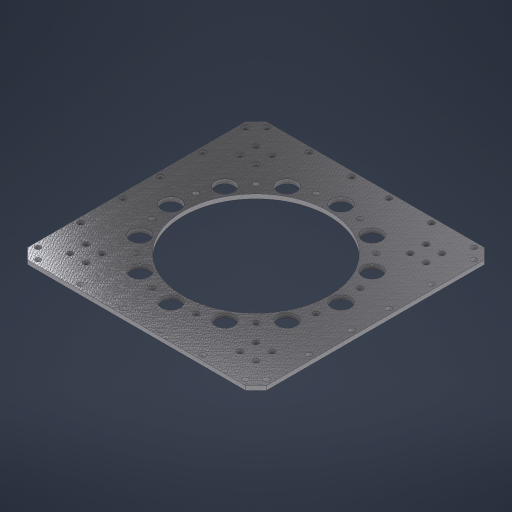
# Autodesk Inventor part: TurretBasePlate
Saved by Autodesk Inventor 2024 (Build 280153000, 153)
## iProperties
Created: 2023-10-18
Part Number: TurretBasePlate
Material: Generic
Document SubType Name: Modeling
Designer: avsar
Density: 1 g/cm^3
Appearance: Machined 02
Author: avsar
Autodesk Inventor part; units mm, degrees
ref_plane "YZ Plane" through (0, 0, 0) normal (1, 0, 0) x (0, 1, 0)
ref_plane "XZ Plane" through (0, 0, 0) normal (0, 1, 0) x (-1, 0, 0)
ref_plane "XY Plane" through (0, 0, 0) normal (0, 0, 1) x (1, 0, 0)
sketch "Sketch1" plane through (0, 0, 0) normal (0, 1, 0) x (-1, 0, 0)
  line L0 (90, 90) -> (-90, 90)
  line L1 (-90, 90) -> (-90, -90)
  line L2 (-90, -90) -> (90, -90)
  line L3 (90, -90) -> (90, 90)
  line L4 (90, 90) -> (-90, -90) construction
  line L5 (-90, 90) -> (90, -90) construction
  point P0 (0, 0)
  dimension "d0" = 180
  dimension "d1" = 180
  constraints: 12 end point, 2 midpoint, 2 parallel, 1 horizontal, 1 perpendicular
  measures "d0" distance of L2.end L1.end
  measures "d1" distance of L1.end L0.end
extrude "Extrusion1" add sketch "Sketch1" along normal mid plane 3.175
sketch "Sketch2" plane through (0, 1.5875, 0) normal (0, 1, 0) x (1, 0, 0)
  line L0 (90, -90) -> (90, 90) construction
  line L1 (90, 90) -> (-90, 90) construction
  line L2 (-90, 90) -> (-90, -90) construction
  line L3 (-90, -90) -> (90, -90) construction
  circle A0 centre (-64, 64) radius 2.5 construction
  line L4 (0, 90) -> (0, -90) construction
  line L5 (-90, 0) -> (90, 0) construction
  circle A1 centre (-58, 58) radius 2
  circle A2 centre (-58, 70) radius 2
  circle A3 centre (-70, 70) radius 2
  circle A4 centre (-70, 58) radius 2
  circle A5 centre (64, 64) radius 2.5 construction
  circle A6 centre (58, 58) radius 2
  circle A7 centre (58, 70) radius 2
  circle A8 centre (70, 70) radius 2
  circle A9 centre (70, 58) radius 2
  circle A10 centre (-64, -64) radius 2.5 construction
  circle A11 centre (-58, -58) radius 2
  circle A12 centre (-58, -70) radius 2
  circle A13 centre (-70, -70) radius 2
  circle A14 centre (-70, -58) radius 2
  circle A15 centre (64, -64) radius 2.5 construction
  circle A16 centre (58, -58) radius 2
  circle A17 centre (58, -70) radius 2
  circle A18 centre (70, -70) radius 2
  circle A19 centre (70, -58) radius 2
  point P0 (0, 0)
  dimension "d4" = 5
  dimension "d5" = 64
  dimension "d6" = 64
  dimension "d7" = 4
  dimension "d8" = 6
  dimension "d9" = 6
  dimension "d12" = 360
  constraints: 20 centre point, 15 symmetric about line, 4 end point, 4 midpoint, 24 other
  measures "d4" diameter of A0
  measures "d5" horizontal distance of point (0, 0) A0.centre
  measures "d6" horizontal distance of point (0, 0) A0.centre
  measures "d7" diameter of A1
  measures "d8" horizontal distance of A1.centre A0.centre
  measures "d9" horizontal distance of A1.centre A0.centre
extrude "Extrusion2" cut sketch "Sketch2" against normal through all
chamfer "Chamfer1" distance 8 angle 45 4 edges at (90, 0, 90) (90, 0, -90) (-90, 0, 90) (-90, 0, -90)
sketch "Sketch3" plane through (0, 1.5875, 0) normal (0, 1, 0) x (1, 0, 0)
  circle A0 centre (0, 0) radius 55
  dimension "d19" = 110
  constraints: 1 centre point, 1 coincident
  measures "d19" diameter of A0
extrude "Extrusion3" cut sketch "Sketch3" against normal through all
sketch "Sketch4" plane through (0, 1.5875, 0) normal (0, 1, 0) x (1, 0, 0)
  circle A0 centre (0, 64) radius 7
  circle A1 centre (-32, 55.4256) radius 7
  circle A2 centre (-55.4256, 32) radius 7
  circle A3 centre (-64, 0) radius 7
  circle A4 centre (-55.4256, -32) radius 7
  circle A5 centre (-32, -55.4256) radius 7
  circle A6 centre (0, -64) radius 7
  circle A7 centre (32, -55.4256) radius 7
  circle A8 centre (55.4256, -32) radius 7
  circle A9 centre (64, 0) radius 7
  circle A10 centre (55.4256, 32) radius 7
  circle A11 centre (32, 55.4256) radius 7
  arc A12 (0, 64) -> (-32, 55.4256) centre (0, 0) ccw
  line L0 (-16.5644, 61.8193) -> (0, 0) construction
  circle A13 centre (-16.5644, 61.8193) radius 2
  circle A14 centre (-45.2548, 45.2548) radius 2
  circle A15 centre (-61.8193, 16.5644) radius 2
  circle A16 centre (-61.8193, -16.5644) radius 2
  circle A17 centre (-45.2548, -45.2548) radius 2
  circle A18 centre (-16.5644, -61.8193) radius 2
  circle A19 centre (16.5644, -61.8193) radius 2
  circle A20 centre (45.2548, -45.2548) radius 2
  circle A21 centre (61.8193, -16.5644) radius 2
  circle A22 centre (61.8193, 16.5644) radius 2
  circle A23 centre (45.2548, 45.2548) radius 2
  circle A24 centre (16.5644, 61.8193) radius 2
  dimension "d23" = 14
  dimension "d24" = 64
  dimension "d27" = 360
  dimension "d31" = 4
  dimension "d34" = 360
  constraints: 25 centre point, 3 point on circle, 2 coincident, 2 end point, 1 vertical alignment, 50 other
  measures "d23" diameter of A0
  measures "d24" distance of point (0, 0) A0.centre
  measures "d31" diameter of A13
extrude "Extrusion5" cut sketch "Sketch4" along normal blind 10 and the other way blind 5
sketch "Sketch8" plane through (0, 1.5875, 0) normal (0, 1, 0) x (1, 0, 0)
  circle A0 centre (-78, -86) radius 2
  line L0 (-90, 82) -> (-90, -82) projected
  line L1 (-82, -90) -> (82, -90) projected
  circle A1 centre (-46, -86) radius 2
  circle A2 centre (-14, -86) radius 2
  circle A3 centre (86, -78) radius 2
  line L2 (90, -82) -> (90, 82) projected
  circle A4 centre (86, -46) radius 2
  circle A5 centre (86, -14) radius 2
  circle A6 centre (78, 86) radius 2
  line L3 (82, 90) -> (-82, 90) projected
  circle A7 centre (46, 86) radius 2
  circle A8 centre (14, 86) radius 2
  circle A9 centre (-86, 78) radius 2
  circle A10 centre (-86, 46) radius 2
  circle A11 centre (-86, 14) radius 2
  circle A12 centre (0, 0) radius 55 construction
  line L4 (0, 55) -> (0, -55) construction
  line L5 (-55, 0) -> (55, 0) construction
  circle A13 centre (78, -86) radius 2
  circle A14 centre (46, -86) radius 2
  circle A15 centre (14, -86) radius 2
  circle A16 centre (86, 78) radius 2
  circle A17 centre (86, 46) radius 2
  circle A18 centre (86, 14) radius 2
  circle A19 centre (-78, 86) radius 2
  circle A20 centre (-46, 86) radius 2
  circle A21 centre (-14, 86) radius 2
  circle A22 centre (-86, -78) radius 2
  circle A23 centre (-86, -46) radius 2
  circle A24 centre (-86, -14) radius 2
  dimension "d63" = 4
  dimension "d65" = 4
  dimension "d68" = 32
  dimension "d73" = 4
  dimension "d74" = 4
  dimension "d75" = 12
  dimension "d78" = 32
  dimension "d85" = 4
  dimension "d86" = 4
  dimension "d87" = 12
  dimension "d90" = 32
  dimension "d97" = 4
  dimension "d98" = 4
  dimension "d99" = 12
  dimension "d102" = 32
  dimension "d109" = 4
  constraints: 24 centre point, 12 symmetric about line, 4 end point, 4 point on circle, 3 vertical, 2 horizontal, 2 midpoint, 1 coincident, 1 perpendicular, 28 other
  measures "d63" diameter of A0
  measures "d65" distance from line of L1 A0.centre
  measures "d68" distance of A0.centre A1.centre
  measures "d73" diameter of A3
  measures "d74" distance from line of L2 A3.centre
  measures "d75" distance from line of L1 A3.centre
  measures "d78" distance of A3.centre A4.centre
  measures "d85" diameter of A6
  measures "d86" distance from line of L3 A6.centre
  measures "d87" distance from line of L2 A6.centre
  measures "d90" distance of A6.centre A7.centre
  measures "d97" diameter of A9
  measures "d98" distance from line of L0 A9.centre
  measures "d99" distance from line of L3 A9.centre
  measures "d102" distance of A9.centre A10.centre
  measures "d109" horizontal distance of L1.start A0.centre
extrude "Extrusion8" cut sketch "Sketch8" against normal through all
body "Solid1"
